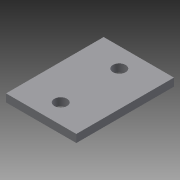
# Autodesk Inventor part: CONNECTOR_PLATE
Saved by Autodesk Inventor 2013 (Build 170138000, 138)
## iProperties
Created: 2013-06-23
Part Number: CONNECTOR_PLATE
Material: Generic
Document SubType Name: Modeling
Designer: Virtual
Density: 1 g/cm^3
Author: Virtual
Autodesk Inventor part; units mm, degrees
ref_plane "YZ Plane" through (0, 0, 0) normal (1, 0, 0) x (0, 1, 0)
ref_plane "XZ Plane" through (0, 0, 0) normal (0, 1, 0) x (-1, 0, 0)
ref_plane "XY Plane" through (0, 0, 0) normal (0, 0, 1) x (1, 0, 0)
sketch "Sketch1" plane through (0, 0, 0) normal (0, 0, 1) x (1, 0, 0)
  line L0 (-9, -12.5) -> (9, -12.5)
  line L1 (9, -12.5) -> (9, 12.5)
  line L2 (9, 12.5) -> (-9, 12.5)
  line L3 (-9, 12.5) -> (-9, -12.5)
  constraints: 8 end point, 2 parallel, 1 horizontal, 1 perpendicular
extrude "Extrusion1" add sketch "Sketch1" along normal blind 2
sketch "Sketch4" plane through (0, 0, 2) normal (0, 0, 1) x (1, 0, 0)
  circle A0 centre (0, 7.5) radius 1.625
  circle A1 centre (0, -7.5) radius 1.625
  point P0 (0, 0)
  dimension "d4" = 3.25
  constraints: 2 centre point
  measures "d4" diameter of A0
hole "Hole1" at (0, -7.5, 2) at (0, 7.5, 2) direction (0, 0, -1) diameter 3.25 end through all
body "Solid1"
